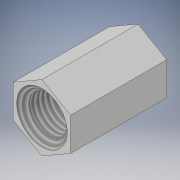
# Autodesk Inventor part: inside thread
Saved by Autodesk Inventor 2017 (Build 210142000, 142)
## iProperties
Created: 2017-01-21
Part Number: inside thread
Material: Generic
Document SubType Name: Modeling
Designer: User
Density: 1 g/cm^3
Appearance: Default
Author: User
Autodesk Inventor part; units mm, degrees
ref_plane "YZ Plane" through (0, 0, 0) normal (1, 0, 0) x (0, 1, 0)
ref_plane "XZ Plane" through (0, 0, 0) normal (0, 1, 0) x (-1, 0, 0)
ref_plane "XY Plane" through (0, 0, 0) normal (0, 0, 1) x (1, 0, 0)
sketch "Sketch1" plane through (0, 0, 0) normal (0, 0, 1) x (1, 0, 0)
  line L0 (0, 12.7583) -> (11.049, 6.3791)
  line L1 (11.049, 6.3791) -> (11.049, -6.3791)
  line L2 (11.049, -6.3791) -> (0, -12.7583)
  line L3 (0, -12.7583) -> (-11.049, -6.3791)
  line L4 (-11.049, -6.3791) -> (-11.049, 6.3791)
  line L5 (-11.049, 6.3791) -> (0, 12.7583)
  point P0 (0, 0)
  point P1 (0, 0)
  dimension "d0" = 22.098
  constraints: 12 end point, 1 coincident, 13 other
  measures "d0" distance between parallel lines of L2 L5
extrude "Extrusion1" add sketch "Sketch1" along normal blind 37.084
sketch "Sketch2" plane through (0, 0, 37.084) normal (0, 0, 1) x (1, 0, 0)
  circle A0 centre (0, 0) radius 7.239
  dimension "d4" = 14.478
  constraints: 1 centre point, 1 coincident
  measures "d4" diameter of A0
extrude "Extrusion2" cut sketch "Sketch2" against normal blind 37.084
chamfer "Chamfer1" distance 2.54 angle 45 1 edges at (-7.239, 0, 37.084)
thread "Thread1" size "1/2-13 UNC" class "2B" standard "ANSI Unified Screw Threads" full length
thread "Thread2" size "3/4" designation "3/4 - 14 NPT" standard "NPT for PVC Pipe and Fitting" full length
body "Solid1"
